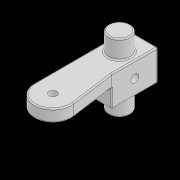
# Autodesk Inventor part: Custom_LeftKnuckle
Saved by Autodesk Inventor 2022 (Build 260153000, 153)
## iProperties
Created: 2022-07-22
Part Number: Custom_LeftKnuckle
Material: Generic
Document SubType Name: Modeling
Designer: tandu
Density: 1 g/cm^3
Appearance: Default
Author: tandu
Autodesk Inventor part; units mm, degrees
ref_plane "YZ Plane" through (0, 0, 0) normal (1, 0, 0) x (0, 1, 0)
ref_plane "XZ Plane" through (0, 0, 0) normal (0, 1, 0) x (-1, 0, 0)
sketch "Sketch1" plane through (0, 0, 0) normal (0, 1, 0) x (-1, 0, 0)
  line L0 (1.27, 1.905) -> (-1.27, 1.905)
  line L1 (-1.27, 1.905) -> (-1.27, -1.905)
  line L2 (-1.27, -1.905) -> (1.27, -1.905)
  line L3 (1.27, -1.905) -> (1.27, 1.905)
  line L4 (1.27, 1.905) -> (-1.27, -1.905) construction
  line L5 (-1.27, 1.905) -> (1.27, -1.905) construction
  circle A0 centre (0, 0) radius 0.889
  line L6 (0, 1.905) -> (0, 5.715) construction
  circle A1 centre (-0.254, 5.715) radius 0.325
  line L7 (1.27, 1.905) -> (1.27, 5.715)
  circle A2 centre (-0.254, 5.715) radius 1.524
  line L8 (-1.27, 1.905) -> (-1.7639, 5.508)
  dimension "d0" = 2.54
  dimension "d1" = 3.81
  dimension "d2" = 1.778
  dimension "d3" = 3.81
  dimension "d4" = 0.65
  dimension "d5" = 3.048
  constraints: 18 end point, 3 centre point, 3 midpoint, 2 coincident, 2 horizontal alignment, 2 parallel, 2 point on circle, 2 vertical, 1 horizontal, 1 perpendicular, 1 tangent
  measures "d0" distance of L2.end L1.end
  measures "d1" distance of L1.end L0.end
  measures "d2" diameter of A0
  measures "d3" distance of L6.start L6.end
  measures "d4" diameter of A1
  measures "d5" diameter of A2
extrude "BaseBoxExtrusion" add sketch "Sketch1" against normal blind 2.54 contours L3 L2 L1 L0 | A0
extrude "NubExtrusion" add sketch "Sketch1" against normal blind 1.016 contours L0 L8 A2 L7 | A2
extrude "TopNub" add sketch "Sketch1" along normal blind 1.524 contours A0
ref_plane "Work Plane1" through (0, -1.27, 0) normal (0, 1, 0) x (1, 0, 0)
mirror "Bottom Nub Mirror1" about plane through (0, -1.27, 0) normal (0, 1, 0) of "TopNub"
sketch "Sketch2" plane through (1.27, -2.54, -1.905) normal (1, 0, 0) x (0, 0, -1)
  line L0 (-3.81, 2.54) -> (0, 2.54) projected
  line L1 (-3.81, 2.54) -> (-3.81, 1.524) projected
  line L2 (-3.81, 1.524) -> (-3.81, 0) projected
  line L3 (0, 0) -> (-3.81, 0) projected
  line L4 (0, 2.54) -> (0, 0) projected
  line L5 (-3.81, 0) -> (0, 0)
  line L6 (0, 0) -> (0, 2.54)
  line L7 (0, 2.54) -> (-3.81, 2.54)
  line L8 (-3.81, 2.54) -> (-3.81, 0)
  line L9 (-3.81, 0) -> (0, 2.54) construction
  line L10 (0, 0) -> (-3.81, 2.54) construction
  circle A0 centre (-1.905, 1.27) radius 0.325
  point P0 (-1.905, 2.54)
  dimension "d12" = 0.65
  constraints: 12 end point, 2 midpoint, 2 parallel, 1 centre point, 1 coincident, 1 horizontal, 1 perpendicular
  measures "d12" diameter of A0
extrude "SideHole" cut sketch "Sketch2" against normal through all contours A0
fillet "Fillet1" radius 0.1 20 edges at (1.27, 0, 0) (1.27, -1.778, 1.905) (1.27, -2.54, 0) (1.27, -1.27, -1.905) (0, 0, -1.905) (-1.27, 0, 1.905) (0.3577, 0, 7.2355) (1.5169, 0, 3.7065) (1.5169, -1.016, 3.7065) (0.3577, -1.016, 7.2355) (-1.27, -1.016, 3.81) (0, -2.54, -1.905) (0, -2.54, 1.905) (-1.27, -2.54, 0) (-1.27, -1.27, -1.905) (-1.27, -1.778, 1.905) (0.889, 0, 0) (0.889, 1.524, 0) (0.889, -2.54, 0) (0.889, -4.064, 0)
ref_plane "Work Plane2" through (0, -1.27, 0) normal (0, 1, 0) x (1, 0, 0)
body "Solid1"
